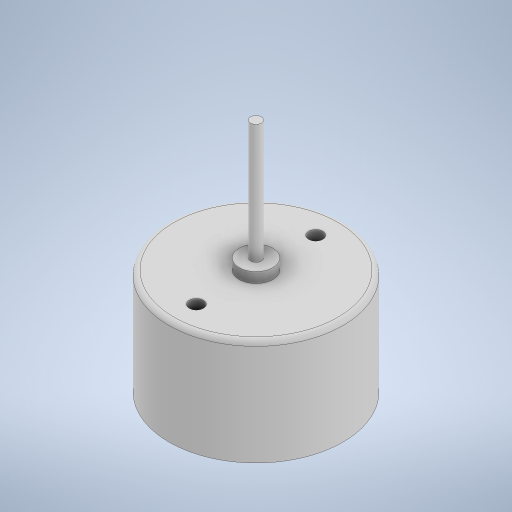
# Autodesk Inventor part: rf500tb
Saved by Autodesk Inventor 2024 (Build 280153000, 153)
## iProperties
Created: 2025-03-10
Part Number: rf500tb
Material: Generic
Document SubType Name: Modeling
Designer: 5454s
Density: 1 g/cm^3
Appearance: Default
Author: 5454s
Autodesk Inventor part; units mm, degrees
ref_plane "YZ Plane" through (0, 0, 0) normal (1, 0, 0) x (0, 1, 0)
ref_plane "XZ Plane" through (0, 0, 0) normal (0, 1, 0) x (-1, 0, 0)
ref_plane "XY Plane" through (0, 0, 0) normal (0, 0, 1) x (1, 0, 0)
sketch "Sketch1" plane through (0, 0, 0) normal (0, 1, 0) x (-1, 0, 0)
  circle A0 centre (0, 0) radius 16
  dimension "d0" = 32
  constraints: 1 centre point, 1 coincident
  measures "d0" diameter of A0
extrude "Extrusion1" add sketch "Sketch1" along normal blind 19.5
sketch "Sketch2" plane through (0, 19.5, 0) normal (0, 1, 0) x (1, 0, 0)
  circle A0 centre (0, 0) radius 16 projected
  circle A1 centre (0, 0) radius 3.1
  dimension "d3" = 6.2
  constraints: 1 centre point, 1 coincident
  measures "d3" diameter of A1
extrude "Extrusion2" add sketch "Sketch2" along normal blind 1.9 contours A1
sketch "Sketch3" plane through (0, 21.4, 0) normal (0, 1, 0) x (1, 0, 0)
  circle A0 centre (0, 0) radius 3.1 projected
  circle A1 centre (0, 0) radius 1
  dimension "d6" = 2
  constraints: 1 centre point, 1 coincident
  measures "d6" diameter of A1
extrude "Extrusion3" add sketch "Sketch3" along normal blind 22 contours A1
sketch "Sketch4" plane through (0, 19.5, 0) normal (0, 1, 0) x (1, 0, 0)
  circle A0 centre (0, 0) radius 3.1 projected
  circle A1 centre (0, 0) radius 16 projected
  circle A2 centre (0, -11) radius 1.3
  circle A3 centre (0, 11) radius 1.3
  line L0 (-16, 0) -> (16, 0)
  dimension "d9" = 2.6
  dimension "d10" = 22
  constraints: 2 centre point, 2 end point, 2 point on circle, 1 equal radius, 1 horizontal, 1 symmetric about line
  measures "d9" diameter of A3
  measures "d10" distance of A3.centre A2.centre
extrude "Extrusion4" cut sketch "Sketch4" against normal blind 4 contours A2 | A3
fillet "Fillet1" radius 0.9 1 edges at (16, 19.5, 0)
body "Solid1"
